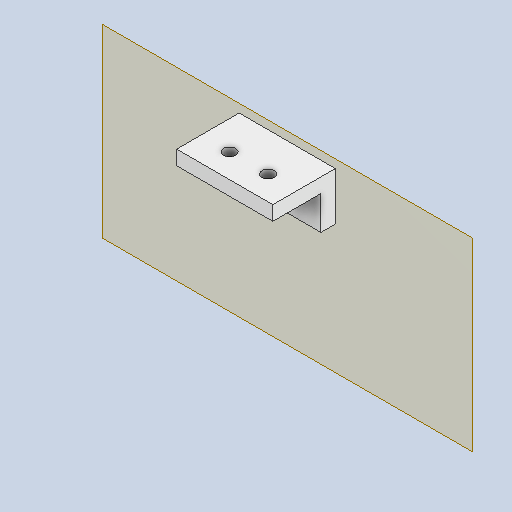
# Autodesk Inventor part: 63
Saved by Autodesk Inventor 2024.3 (Build 283343000, 343)
## iProperties
Created: 2024-09-09
Part Number: 63
Material: LCP 플라스틱
Document SubType Name: Modeling
Designer: 구지현
Density: 1.626 g/cm^3
Appearance: 매끄러움 - 흰색
Author: 구지현
Autodesk Inventor part; units mm, degrees
ref_plane "YZ Plane" through (0, 0, 0) normal (1, 0, 0) x (0, 1, 0)
ref_plane "XZ Plane" through (0, 0, 0) normal (0, 1, 0) x (-1, 0, 0)
ref_plane "XY Plane" through (0, 0, 0) normal (0, 0, 1) x (1, 0, 0)
ref_plane "작업 평면1" through (0, 0, 0) normal (0, 0, 1) x (1, 0, 0)
sketch "스케치1" plane through (0, 0, 0) normal (0, 0, 1) x (1, 0, 0)
  line L0 (-35, -17.5) -> (35, -17.5) projected
  line L1 (35, -17.5) -> (35, 17.5) projected
  line L2 (35, 17.5) -> (-35, 17.5) projected
  line L3 (-35, 17.5) -> (-35, -17.5) projected
  line L4 (35, -17.5) -> (-35, -17.5) projected
  line L5 (-35, -17.5) -> (-35, -23.5) projected
  line L6 (35, -23.5) -> (-35, -23.5) projected
  line L7 (35, -17.5) -> (35, -23.5) projected
  line L8 (35, 0) -> (10, 0)
  line L9 (-35, 0) -> (-10, 0)
  line L10 (10, 0) -> (-10, 0)
  line L11 (10, 0) -> (10, 17.5)
  line L12 (-10, 0) -> (-10, 17.5)
  line L13 (10, 17.5) -> (-10, 17.5)
  line L14 (-10, 17.5) -> (-10, 7.5)
  line L15 (-10, 7.5) -> (10, 7.5)
  line L16 (10, 7.5) -> (10, 17.5)
  point P0 (0, 0)
  dimension "d0" = 25
  dimension "d1" = 25
  dimension "d2" = 20
  dimension "d3" = 10
  constraints: 18 end point, 3 horizontal, 3 perpendicular, 3 point on line, 2 midpoint, 2 parallel, 1 collinear
  measures "d0" distance of L8.start L8.end
  measures "d1" distance of L9.start L9.end
  measures "d2" distance of L8.end L9.end
  measures "d3" distance of L14.end L13.end
extrude "돌출1" add sketch "스케치1" along normal blind 3 contours L2 L11 L15 L12
sketch "스케치2" plane through (0, 0, 3) normal (0, 0, 1) x (1, 0, 0)
  line L0 (10, 7.5) -> (10, 17.5) projected
  line L1 (10, 17.5) -> (-10, 17.5) projected
  line L2 (-10, 17.5) -> (-10, 7.5) projected
  line L3 (-10, 7.5) -> (10, 7.5) projected
  line L4 (10, 17.5) -> (-10, 17.5)
  line L5 (-10, 17.5) -> (-10, 14.5)
  line L6 (-10, 14.5) -> (10, 14.5)
  line L7 (10, 14.5) -> (10, 17.5)
  point P0 (0, 0)
  point P1 (10, 14.5)
  dimension "d6" = 3
  constraints: 8 end point, 2 parallel, 1 horizontal, 1 perpendicular, 1 point on line
  measures "d6" distance of L5.end L4.end
extrude "돌출2" add sketch "스케치2" along normal blind 10 contours L6 L2 L1 L0
sketch "스케치3" plane through (0, 0, 3) normal (0, 0, 1) x (1, 0, 0)
  line L0 (10, 14.5) -> (-10, 14.5) projected
  line L1 (-10, 14.5) -> (-10, 7.5) projected
  line L2 (-10, 7.5) -> (10, 7.5) projected
  line L3 (10, 7.5) -> (10, 14.5) projected
  line L4 (10, 11) -> (4, 11)
  line L5 (-10, 11) -> (-4, 11)
  circle A0 centre (4, 11) radius 1.25
  circle A1 centre (-4, 11) radius 1.25
  point P0 (0, 0)
  dimension "d9" = 6
  dimension "d10" = 6
  dimension "d11" = 2.5
  dimension "d12" = 2.5
  constraints: 4 end point, 2 centre point, 2 coincident, 2 horizontal, 2 midpoint
  measures "d9" distance of L4.start L4.end
  measures "d10" distance of L5.start L5.end
  measures "d11" diameter of A0
  measures "d12" diameter of A1
extrude "돌출3" cut sketch "스케치3" against normal blind 10 contours A0 | A1
sketch "스케치4" plane through (-10, 14.5, 3) normal (0, -1, 0) x (1, 0, 0)
  line L0 (20, 0) -> (0, 0) projected
  line L1 (20, 0) -> (20, 10) projected
  line L2 (0, 10) -> (20, 10) projected
  line L3 (0, 0) -> (0, 10) projected
  line L4 (20, 5) -> (14, 5)
  line L5 (0, 5) -> (6, 5)
  circle A0 centre (14, 5) radius 1.25
  circle A1 centre (6, 5) radius 1.25
  point P0 (10, -3)
  dimension "d15" = 6
  dimension "d16" = 6
  dimension "d17" = 2.5
  dimension "d18" = 2.5
  constraints: 4 end point, 2 centre point, 2 coincident, 2 horizontal, 2 midpoint
  measures "d15" distance of L4.start L4.end
  measures "d16" distance of L5.start L5.end
  measures "d17" diameter of A0
  measures "d18" diameter of A1
extrude "돌출4" cut sketch "스케치4" against normal blind 10 contours A0 | A1
